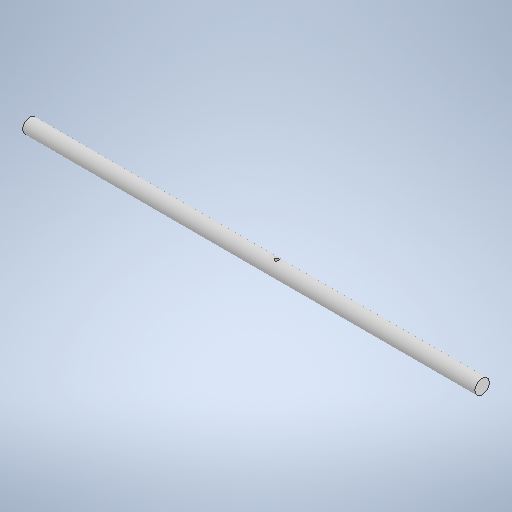
# Autodesk Inventor part: stationaryrod
Saved by Autodesk Inventor 2025.1 (Build 291241000, 241)
## iProperties
Created: 2025-11-11
Part Number: stationaryrod
Material: Generic
Document SubType Name: Modeling
Designer: mukund
Density: 1 g/cm^3
Appearance: Default
Author: mukund
Autodesk Inventor part; units mm, degrees
ref_plane "YZ Plane" through (0, 0, 0) normal (1, 0, 0) x (0, 1, 0)
ref_plane "XZ Plane" through (0, 0, 0) normal (0, 1, 0) x (-1, 0, 0)
ref_plane "XY Plane" through (0, 0, 0) normal (0, 0, 1) x (1, 0, 0)
sketch "Sketch1" plane through (0, 0, 0) normal (0, 1, 0) x (-1, 0, 0)
  line L0 (0, 0) -> (-18, 0)
  circle A0 centre (-18, 0) radius 1.6
  dimension "d12" = 18
  dimension "d13" = 3.2
  constraints: 2 end point, 1 centre point, 1 coincident, 1 horizontal
  measures "d12" distance of L0.start L0.end
  measures "d13" diameter of A0
sketch "Sketch2" plane through (0, 0, 0) normal (1, 0, 0) x (0, 1, 0)
  circle A0 centre (0, 0) radius 6.35
  dimension "d1" = 12.7
  constraints: 1 centre point, 1 coincident
  measures "d1" diameter of A0
extrude "Extrusion1" add sketch "Sketch2" along normal mid plane 395
extrude "Extrusion3" cut sketch "Sketch1" along normal mid plane 30
body "Solid1"
